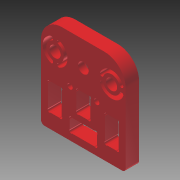
# Autodesk Inventor part: gantry1
Saved by Autodesk Inventor 2012 SP1 (Build 160190100, 190)
## iProperties
Created: 2011-10-14
Part Number: gantry1
Document SubType Name: Modeling
Designer: cramera
Density: 0.952 g/cm^3
Material: High Density Polyethylene
Mass: 49.0795 g
Surface Area: 206.871 cm^2
Volume: 51.5541 cm^3
Autodesk Inventor part; units mm, degrees
ref_plane "YZ Plane" through (0, 0, 0) normal (1, 0, 0) x (0, 1, 0)
ref_plane "XZ Plane" through (0, 0, 0) normal (0, 1, 0) x (-1, 0, 0)
ref_plane "XY Plane" through (0, 0, 0) normal (0, 0, 1) x (1, 0, 0)
derived "skeleton.ipt"
sketch "POCKET_1-4" plane through (0, 0, 0) normal (0, 0, 1) x (1, 0, 0)
  arc A0 (371.8465, 703.1072) -> (359.1465, 690.4072) centre (371.8465, 690.4072) ccw
  arc A1 (359.1465, 690.4072) -> (371.8465, 677.7072) centre (371.8465, 690.4072) ccw
  arc A2 (371.8465, 677.7072) -> (384.5465, 690.4072) centre (371.8465, 690.4072) ccw
  arc A3 (384.5465, 690.4072) -> (371.8465, 703.1072) centre (371.8465, 690.4072) ccw
  constraints: 8 point on circle, 4 centre point
sketch "STOCK_12MM" plane through (0, 0, 0) normal (0, 0, 1) x (1, 0, 0)
  line L0 (457.2, 914.4) -> (457.2, 0)
  line L1 (457.2, 0) -> (914.4, 0)
  line L2 (914.4, 0) -> (914.4, 914.4)
  line L3 (914.4, 914.4) -> (457.2, 914.4)
  line L4 (0, 0) -> (457.2, 0)
  line L5 (457.2, 0) -> (457.2, 914.4)
  line L6 (457.2, 914.4) -> (0, 914.4)
  line L7 (0, 914.4) -> (0, 0)
  constraints: 16 end point
sketch "THROUGH-CUT" plane through (0, 0, 0) normal (0, 0, 1) x (1, 0, 0)
  line L0 (391.2775, 663.0479) -> (391.2775, 643.154)
  circle A0 centre (346.4465, 690.4072) radius 5
  arc A1 (367.084, 690.4072) -> (371.8465, 685.6447) centre (371.8465, 690.4072) ccw
  arc A2 (371.8465, 685.6447) -> (376.609, 690.4072) centre (371.8465, 690.4072) ccw
  arc A3 (376.609, 690.4072) -> (371.8465, 695.1697) centre (371.8465, 690.4072) ccw
  arc A4 (371.8465, 695.1697) -> (367.084, 690.4072) centre (371.8465, 690.4072) ccw
  arc A5 (383.848, 672.5635) -> (381.435, 670.1505) centre (383.848, 670.1505) ccw
  arc A6 (381.435, 670.1505) -> (383.848, 667.7375) centre (383.848, 670.1505) ccw
  arc A7 (383.848, 667.7375) -> (386.261, 670.1505) centre (383.848, 670.1505) ccw
  arc A8 (386.261, 670.1505) -> (383.848, 672.5635) centre (383.848, 670.1505) ccw
  arc A9 (340.0965, 643.154) -> (342.3415, 640.909) centre (341.219, 642.0315) ccw
  line L1 (342.3415, 640.909) -> (350.1704, 640.909)
  arc A10 (350.1704, 640.909) -> (352.4155, 643.154) centre (351.2929, 642.0315) ccw
  line L2 (352.4155, 643.154) -> (352.4155, 663.0479)
  arc A11 (352.4155, 663.0479) -> (350.1704, 665.293) centre (351.2929, 664.1704) ccw
  line L3 (350.1704, 665.293) -> (342.3415, 665.293)
  arc A12 (342.3415, 665.293) -> (340.0965, 663.0479) centre (341.219, 664.1704) ccw
  line L4 (340.0965, 663.0479) -> (340.0965, 643.154)
  arc A13 (365.687, 654.2983) -> (367.932, 652.0532) centre (366.8095, 653.1758) ccw
  line L5 (367.932, 652.0532) -> (375.7609, 652.0532)
  arc A14 (375.7609, 652.0532) -> (378.006, 654.2983) centre (376.8834, 653.1758) ccw
  line L6 (378.006, 654.2983) -> (378.006, 669.1122)
  arc A15 (378.006, 669.1122) -> (375.7609, 671.3572) centre (376.8834, 670.2347) ccw
  line L7 (375.7609, 671.3572) -> (367.932, 671.3572)
  arc A16 (367.932, 671.3572) -> (365.687, 669.1122) centre (366.8095, 670.2347) ccw
  line L8 (365.687, 669.1122) -> (365.687, 654.2983)
  arc A17 (333.7465, 631.1605) -> (336.9215, 627.9855) centre (336.9215, 631.1605) ccw
  line L9 (336.9215, 627.9855) -> (406.7715, 627.9855)
  arc A18 (406.7715, 627.9855) -> (409.9465, 631.1605) centre (406.7715, 631.1605) ccw
  line L10 (409.9465, 631.1605) -> (409.9465, 693.5822)
  line L11 (390.8965, 712.6322) -> (352.7965, 712.6322)
  arc A19 (352.7965, 712.6322) -> (333.7465, 693.5822) centre (352.7965, 693.5822) ccw
  line L12 (333.7465, 693.5822) -> (333.7465, 631.1605)
  arc A20 (359.845, 672.5635) -> (357.432, 670.1505) centre (359.845, 670.1505) ccw
  arc A21 (357.432, 670.1505) -> (359.845, 667.7375) centre (359.845, 670.1505) ccw
  arc A22 (359.845, 667.7375) -> (362.258, 670.1505) centre (359.845, 670.1505) ccw
  arc A23 (362.258, 670.1505) -> (359.845, 672.5635) centre (359.845, 670.1505) ccw
  arc A24 (409.9465, 693.5822) -> (390.8965, 712.6322) centre (390.8965, 693.5822) ccw
  line L13 (361.8995, 634.3355) -> (381.7934, 634.3355)
  arc A25 (381.7934, 634.3355) -> (384.0385, 636.5805) centre (382.9159, 635.458) ccw
  line L14 (384.0385, 636.5805) -> (384.0385, 644.4094)
  arc A26 (384.0385, 644.4094) -> (381.7934, 646.6545) centre (382.9159, 645.5319) ccw
  line L15 (381.7934, 646.6545) -> (361.8995, 646.6545)
  arc A27 (361.8995, 646.6545) -> (359.6545, 644.4094) centre (360.777, 645.5319) ccw
  line L16 (359.6545, 644.4094) -> (359.6545, 636.5805)
  circle A28 centre (397.2465, 690.4072) radius 5
  arc A29 (391.2775, 643.154) -> (393.5225, 640.909) centre (392.4, 642.0315) ccw
  line L17 (393.5225, 640.909) -> (401.3514, 640.909)
  arc A30 (401.3514, 640.909) -> (403.5965, 643.154) centre (402.4739, 642.0315) ccw
  arc A31 (359.6545, 636.5805) -> (361.8995, 634.3355) centre (360.777, 635.458) ccw
  line L18 (403.5965, 643.154) -> (403.5965, 663.0479)
  arc A32 (403.5965, 663.0479) -> (401.3514, 665.293) centre (402.4739, 664.1704) ccw
  line L19 (401.3514, 665.293) -> (393.5225, 665.293)
  arc A33 (393.5225, 665.293) -> (391.2775, 663.0479) centre (392.4, 664.1704) ccw
  arc A34 (406.1219, 688.68) -> (404.6347, 687.6479) centre (406.1219, 687.0925) ccw
  arc A35 (389.8582, 687.6479) -> (404.6347, 687.6479) centre (397.2465, 690.4072) ccw
  arc A36 (389.8582, 687.6479) -> (388.371, 688.68) centre (388.371, 687.0925) ccw
  line L20 (388.371, 688.68) -> (388.2627, 688.68)
  arc A37 (388.2627, 688.68) -> (386.7733, 686.543) centre (388.2627, 687.0925) ccw
  arc A38 (386.7733, 686.543) -> (407.7196, 686.543) centre (397.2465, 690.4072) ccw
  arc A39 (407.7196, 686.543) -> (406.2303, 688.68) centre (406.2303, 687.0925) ccw
  line L21 (406.2303, 688.68) -> (406.1219, 688.68)
  arc A40 (386.7733, 694.2714) -> (388.2627, 692.1344) centre (388.2627, 693.7219) ccw
  arc A41 (407.7196, 694.2714) -> (386.7733, 694.2714) centre (397.2465, 690.4072) ccw
  arc A42 (406.2303, 692.1344) -> (407.7196, 694.2714) centre (406.2303, 693.7219) ccw
  line L22 (406.2303, 692.1344) -> (406.1219, 692.1344)
  arc A43 (404.6347, 693.1665) -> (406.1219, 692.1344) centre (406.1219, 693.7219) ccw
  arc A44 (404.6347, 693.1665) -> (389.8582, 693.1665) centre (397.2465, 690.4072) ccw
  arc A45 (388.371, 692.1344) -> (389.8582, 693.1665) centre (388.371, 693.7219) ccw
  line L23 (388.371, 692.1344) -> (388.2627, 692.1344)
  arc A46 (344.7193, 681.5318) -> (343.6872, 683.019) centre (343.1318, 681.5318) ccw
  line L24 (344.7193, 681.5318) -> (344.7193, 681.4234)
  arc A47 (342.5823, 679.9341) -> (344.7193, 681.4234) centre (343.1318, 681.4234) ccw
  arc A48 (342.5823, 700.8804) -> (342.5823, 679.9341) centre (346.4465, 690.4072) ccw
  arc A49 (344.7193, 699.391) -> (342.5823, 700.8804) centre (343.1318, 699.391) ccw
  line L25 (344.7193, 699.391) -> (344.7193, 699.2827)
  arc A50 (343.6872, 697.7955) -> (344.7193, 699.2827) centre (343.1318, 699.2827) ccw
  arc A51 (343.6872, 697.7955) -> (343.6872, 683.019) centre (346.4465, 690.4072) ccw
  arc A52 (348.1737, 699.2827) -> (349.2058, 697.7955) centre (349.7612, 699.2827) ccw
  arc A53 (349.2058, 683.019) -> (349.2058, 697.7955) centre (346.4465, 690.4072) ccw
  arc A54 (349.2058, 683.019) -> (348.1737, 681.5318) centre (349.7612, 681.5318) ccw
  line L26 (348.1737, 681.5318) -> (348.1737, 681.4234)
  arc A55 (348.1737, 681.4234) -> (350.3107, 679.9341) centre (349.7612, 681.4234) ccw
  arc A56 (350.3107, 679.9341) -> (350.3107, 700.8804) centre (346.4465, 690.4072) ccw
  arc A57 (350.3107, 700.8804) -> (348.1737, 699.391) centre (349.7612, 699.391) ccw
  line L27 (348.1737, 699.391) -> (348.1737, 699.2827)
  dimension "d5" = 10
  dimension "d6" = 10
  constraints: 112 point on circle, 58 centre point, 56 end point
  measures "d5" diameter of A0
  measures "d6" diameter of A28
extrude "Extrusion1" add sketch "THROUGH-CUT" along normal blind 12
extrude "Extrusion2" cut sketch "POCKET_1-4" along normal blind 6.35
equation "\"d6\" = d5"
equation "\"d1\" = StockThickness"
equation "\"StockThickness\" = 12"
body "Solid1"
